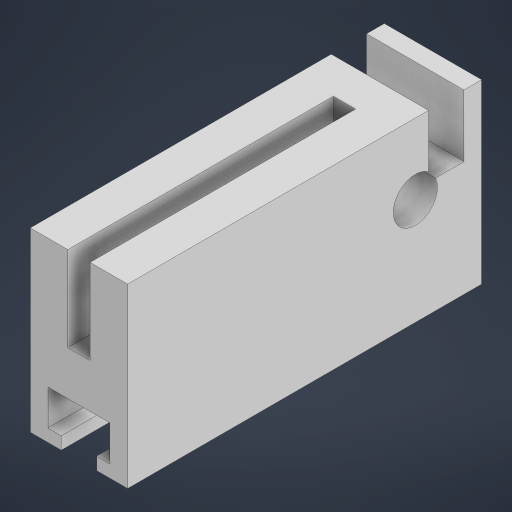
# Autodesk Inventor part: Drone_Launcher_Carriage
Saved by Autodesk Inventor 2023 (Build 270158000, 158)
## iProperties
Created: 2024-02-18
Part Number: Drone_Launcher_Carriage
Material: Generic
Document SubType Name: Modeling
Designer: kelle
Density: 1 g/cm^3
Appearance: Default
Author: kelle
Autodesk Inventor part; units mm, degrees
ref_plane "YZ Plane" through (0, 0, 0) normal (1, 0, 0) x (0, 1, 0)
ref_plane "XZ Plane" through (0, 0, 0) normal (0, 1, 0) x (-1, 0, 0)
ref_plane "XY Plane" through (0, 0, 0) normal (0, 0, 1) x (1, 0, 0)
sketch "Sketch1" plane through (0, 0, 0) normal (0, 0, 1) x (1, 0, 0)
  line L0 (2.54, -4.344) -> (-2.54, -4.344)
  line L1 (-2.54, -4.344) -> (-2.54, 4.344)
  line L2 (-2.54, 4.344) -> (2.54, 4.344)
  line L3 (2.54, 4.344) -> (2.54, -4.344)
  line L4 (2.54, -4.344) -> (-2.54, 4.344) construction
  line L5 (-2.54, -4.344) -> (2.54, 4.344) construction
  line L6 (4.445, 6.884) -> (-4.445, 6.884)
  line L7 (-4.445, 6.884) -> (-4.445, 1.804)
  line L8 (-4.445, 1.804) -> (4.445, 1.804)
  line L9 (4.445, 1.804) -> (4.445, 6.884)
  line L10 (4.445, 6.884) -> (-4.445, 1.804) construction
  line L11 (-4.445, 6.884) -> (4.445, 1.804) construction
  line L12 (3.8177, 1.5502) -> (-3.8177, 7.1379) construction
  line L13 (-4.445, -1.73) -> (4.445, 10.418) construction
  line L14 (6.985, 0) -> (-6.985, 0)
  line L15 (-6.985, 0) -> (-6.985, 25.4)
  line L16 (-6.985, 25.4) -> (6.985, 25.4)
  line L17 (6.985, 25.4) -> (6.985, 0)
  line L18 (6.985, 0) -> (-6.985, 25.4) construction
  line L19 (-6.985, 0) -> (6.985, 25.4) construction
  line L20 (0, 25.4) -> (0, 0) construction
  line L21 (-1.5875, 25.4) -> (1.5875, 25.4)
  line L22 (1.5875, 25.4) -> (1.5875, 13.234)
  line L23 (1.5875, 13.234) -> (-1.5875, 13.234)
  line L24 (-1.5875, 13.234) -> (-1.5875, 25.4)
  point P0 (0, 4.344)
  point P1 (0, 12.7)
  point P2 (2.54, 1.804)
  point P3 (2.54, 0)
  point P4 (-2.54, 0)
  point P5 (-2.54, 1.804)
  dimension "d0" = 5.08
  dimension "d1" = 8.89
  dimension "d2" = 5.08
  dimension "d3" = 8.89
  dimension "d4" = 8.89
  dimension "d5" = 13.97
  dimension "d6" = 25.4
  dimension "d7" = 0
  dimension "d8" = 3.175
  dimension "d9" = 1.5875
  dimension "d27" = 6.35
  constraints: 50 end point, 10 midpoint, 8 parallel, 4 horizontal, 4 perpendicular, 1 point on line
  measures "d0" distance of L1.end L2.end
  measures "d1" distance of L8.end L7.end
  measures "d2" distance of L7.end L6.end
  measures "d3" distance of L12.end L13.end
  measures "d4" distance of L13.start L12.end
  measures "d5" distance of L15.end L16.end
  measures "d6" distance of L14.end L15.end
  measures "d7" distance from line of L20.end L14
  measures "d8" distance of L22.end L23.end
  measures "d9" distance between parallel lines of L20 L22
  measures "d27" distance between parallel lines of L6 L23
extrude "Extrusion1" add sketch "Sketch1" along normal blind 44.45 contours L3 L8 L9 L6 L7 L1 L14 L15 L16 L24 L23 L22 L17
sketch "Sketch2" plane through (0, 0, 0) normal (0, 0, -1) x (-1, 0, 0)
  line L0 (4.445, 6.884) -> (-4.445, 6.884) projected
  line L1 (4.445, 1.804) -> (4.445, 6.884) projected
  line L2 (2.54, 1.804) -> (4.445, 1.804) projected
  line L3 (2.54, 0) -> (2.54, 1.804) projected
  line L4 (6.985, 0) -> (2.54, 0) projected
  line L5 (6.985, 25.4) -> (6.985, 0) projected
  line L6 (1.5875, 25.4) -> (6.985, 25.4) projected
  line L7 (1.5875, 13.234) -> (1.5875, 25.4) projected
  line L8 (-1.5875, 13.234) -> (1.5875, 13.234) projected
  line L9 (-1.5875, 25.4) -> (-1.5875, 13.234) projected
  line L10 (-6.985, 25.4) -> (-1.5875, 25.4) projected
  line L11 (-6.985, 0) -> (-6.985, 25.4) projected
  line L12 (-2.54, 0) -> (-6.985, 0) projected
  line L13 (-2.54, 1.804) -> (-2.54, 0) projected
  line L14 (-4.445, 1.804) -> (-2.54, 1.804) projected
  line L15 (-4.445, 6.884) -> (-4.445, 1.804) projected
  line L16 (-1.5875, 25.4) -> (1.5875, 25.4)
  line L17 (1.5875, 25.4) -> (1.5875, 13.234)
  line L18 (1.5875, 13.234) -> (-1.5875, 13.234)
  line L19 (-1.5875, 13.234) -> (-1.5875, 25.4)
  point P0 (0, 0)
  point P1 (1.5875, 25.4)
  constraints: 8 end point, 2 parallel, 1 horizontal, 1 perpendicular
extrude "Extrusion2" add sketch "Sketch2" against normal blind 6.35 contours L7 L8 L9 L16
sketch "Sketch3" plane through (6.985, 0, 0) normal (1, 0, 0) x (0, 0, -1)
  line L0 (0, 0) -> (0, 25.4) projected
  line L1 (0, 25.4) -> (-44.45, 25.4) projected
  line L2 (-44.45, 0) -> (-44.45, 25.4) projected
  line L3 (0, 0) -> (-44.45, 0) projected
  line L4 (-6.35, 25.4) -> (-6.35, 13.234) projected
  circle A0 centre (-3.175, 15.24) radius 3.175
  point P0 (0, 0)
  point P1 (0, 12.7)
  dimension "d14" = 6.35
  dimension "d15" = 3.175
  dimension "d16" = 10.16
  constraints: 1 centre point, 1 midpoint
  measures "d14" diameter of A0
  measures "d15" horizontal distance of point (0, 12.7) A0.centre
  measures "d16" distance from line of L1 A0.centre
extrude "Extrusion3" cut sketch "Sketch3" against normal through all contours A0
sketch "Sketch4" plane through (0, 0, 0) normal (0, 0, -1) x (-1, 0, 0)
  line L0 (4.445, 6.884) -> (-4.445, 6.884) projected
  line L1 (4.445, 1.804) -> (4.445, 6.884) projected
  line L2 (2.54, 1.804) -> (4.445, 1.804) projected
  line L3 (2.54, 0) -> (2.54, 1.804) projected
  line L4 (6.985, 0) -> (2.54, 0) projected
  line L5 (6.985, 25.4) -> (6.985, 15.24) projected
  line L6 (-6.985, 25.4) -> (6.985, 25.4) projected
  line L7 (-6.985, 0) -> (-6.985, 15.24) projected
  line L8 (-2.54, 0) -> (-6.985, 0) projected
  line L9 (-2.54, 1.804) -> (-2.54, 0) projected
  line L10 (-4.445, 1.804) -> (-2.54, 1.804) projected
  line L11 (-4.445, 6.884) -> (-4.445, 1.804) projected
  line L12 (-6.985, 0) -> (-6.985, 25.4) projected
  line L13 (-6.985, 12.7) -> (6.985, 12.7)
  line L14 (6.985, 25.4) -> (6.985, 0) projected
  line L15 (-6.985, 15.24) -> (6.985, 15.24) projected
  line L16 (-6.985, 15.24) -> (-6.985, 25.4) projected
  line L17 (6.985, 15.24) -> (6.985, 0) projected
  point P0 (0, 0)
  point P1 (-6.985, 12.7)
  point P2 (6.985, 12.7)
  dimension "d19" = 12.7
  constraints: 2 end point, 2 midpoint, 1 perpendicular
  measures "d19" distance between parallel lines of L6 L13
extrude "Extrusion4" add sketch "Sketch4" along normal blind 6.35
sketch "Sketch5" plane through (-6.985, 25.4, 44.45) normal (0, 1, 0) x (1, 0, 0)
  line L0 (0, 50.8) -> (0, 0) projected
  line L1 (13.97, 50.8) -> (13.97, 0) projected
  line L2 (0, 50.8) -> (13.97, 50.8)
  line L3 (13.97, 50.8) -> (13.97, 40.64)
  line L4 (13.97, 40.64) -> (0, 40.64)
  line L5 (0, 40.64) -> (0, 50.8)
  line L6 (0, 48.26) -> (13.97, 48.26)
  line L7 (13.97, 48.26) -> (13.97, 43.18)
  line L8 (13.97, 43.18) -> (0, 43.18)
  line L9 (0, 43.18) -> (0, 48.26)
  line L10 (0, 48.26) -> (13.97, 43.18) construction
  line L11 (13.97, 48.26) -> (0, 43.18) construction
  point P0 (6.985, 44.45)
  point P1 (6.985, 45.72)
  point P2 (0, 43.18)
  dimension "d22" = 10.16
  dimension "d23" = 5.08
  dimension "d24" = 5.08
  dimension "d29" = 0
  constraints: 20 end point, 4 parallel, 2 horizontal, 2 midpoint, 2 perpendicular, 2 point on line
  measures "d22" distance of L2.end L3.end
  measures "d23" distance of L6.end L7.end
  measures "d24" distance from line of L4 point (6.985, 45.72)
  measures "d29" distance between parallel lines of L0 L9
extrude "Extrusion5" cut sketch "Sketch5" against normal blind 8.89 contours L6 L1 L8 L0
fillet "Fillet1" [suppressed]
body "Solid1"
